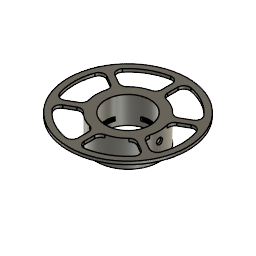
Font Reel (Autodesk Fusion 360 design; units mm, degrees)
part number: 2026-01-12-12-34-36-869
Autodesk Fusion 360 part; units mm, degrees
sketch "Sketch1" plane through (0, 0, 0) normal (0, 0, 1) x (1, 0, 0)
  circle A0 centre (0, 0) radius 90
  circle A1 centre (0, 0) radius 50
  circle A2 centre (0, 0) radius 53
  circle A3 centre (0, 0) radius 100
  line L0 (-5, 89.861) -> (-5, 52.7636)
  line L1 (5, 89.861) -> (5, 52.7636)
  line L2 (0, 110) -> (0, -110)
  line L3 (-80.3219, 40.6004) -> (-48.1946, 22.0517)
  line L4 (-75.3219, 49.2606) -> (-43.1946, 30.7119)
  line L5 (-75.3219, -49.2606) -> (-43.1946, -30.7119)
  line L6 (-80.3219, -40.6004) -> (-48.1946, -22.0517)
  line L7 (5, -89.861) -> (5, -52.7636)
  line L8 (-5, -89.861) -> (-5, -52.7636)
  line L9 (80.3219, -40.6004) -> (48.1946, -22.0517)
  line L10 (75.3219, -49.2606) -> (43.1946, -30.7119)
  line L11 (75.3219, 49.2606) -> (43.1946, 30.7119)
  line L12 (80.3219, 40.6004) -> (48.1946, 22.0517)
  circle A4 centre (0, 0) radius 40
  line L13 (-1.5, 49.9775) -> (-1.5, 39.9719)
  line L14 (1.5, 49.9775) -> (1.5, 39.9719)
  line L15 (-42.5318, 26.2878) -> (-33.8667, 21.285)
  line L16 (-44.0318, 23.6897) -> (-35.3667, 18.6869)
  line L17 (-44.0318, -23.6897) -> (-35.3667, -18.6869)
  line L18 (-42.5318, -26.2878) -> (-33.8667, -21.285)
  line L19 (-1.5, -49.9775) -> (-1.5, -39.9719)
  line L20 (1.5, -49.9775) -> (1.5, -39.9719)
  line L21 (42.5318, -26.2878) -> (33.8667, -21.285)
  line L22 (44.0318, -23.6897) -> (35.3667, -18.6869)
  line L23 (44.0318, 23.6897) -> (35.3667, 18.6869)
  line L24 (42.5318, 26.2878) -> (33.8667, 21.285)
  circle A5 centre (0, 0) radius 47
  circle A6 centre (0, 0) radius 37
  circle A7 centre (0, 0) radius 35.5
  line L25 (12.1417, 33.3591) -> (0, 0)
  line L26 (-12.1417, 33.3591) -> (0, 0)
  line L27 (12.1417, 33.3591) -> (12.6547, 34.7686)
  line L28 (-12.1417, 33.3591) -> (-12.6547, 34.7686)
  line L29 (-33.3591, 12.1417) -> (-34.7686, 12.6547)
  line L30 (-33.3591, -12.1417) -> (-34.7686, -12.6547)
  line L31 (-12.1417, -33.3591) -> (-12.6547, -34.7686)
  line L32 (12.1417, -33.3591) -> (12.6547, -34.7686)
  line L33 (33.3591, -12.1417) -> (34.7686, -12.6547)
  line L34 (33.3591, 12.1417) -> (34.7686, 12.6547)
  line L35 (-10.1986, 35.5667) -> (-9.7851, 34.1248)
  line L36 (-9.7851, 34.1248) -> (0, 0)
  line L37 (-35.5667, -10.1986) -> (-34.1248, -9.7851)
  line L38 (10.1986, -35.5667) -> (9.7851, -34.1248)
  line L39 (35.5667, 10.1986) -> (34.1248, 9.7851)
  dimension "d1" = 180
  dimension "d2" = 100
  dimension "d3" = 3
  dimension "d8" = 10
  dimension "d9" = 10
  dimension "d11" = 360
  dimension "d18" = -10
  dimension "d19" = 3
  dimension "d21" = 360
  dimension "d24" = -3
  dimension "d28" = -3
  dimension "d44" = -1.5
  dimension "d47" = 40
  dimension "d48" = 20
  dimension "d50" = 360
  dimension "d54" = 4
  dimension "d56" = 360
  constraint coincident A0.centre A1.centre
  constraint concentric A0 A1
  constraint coincident A0 L0.start
  constraint coincident A2 L0.end
  constraint vertical L0
  constraint coincident A0 L1.start
  constraint coincident A2 L1.end
  constraint parallel L0 L1
  constraint vertical L2
  constraint symmetric L0 L1 L2
  constraint coincident L2 A0.centre
  constraint coincident A1 L13.start
  constraint coincident A4 L13.end
  constraint parallel L2 L13
  constraint coincident A1 L14.start
  constraint coincident A4 L14.end
  constraint parallel L2 L14
  constraint symmetric L2 L13 L14
  constraint coincident A7 L25.start
  constraint coincident A7 L26.start
  constraint coincident A6 L27.end
  constraint parallel L25 L27
  constraint coincident A6 L28.end
  constraint parallel L26 L28
  constraint coincident A6 L35.start
  constraint coincident A7 L35.end
  measures "d1" diameter of A0
  measures "d2" diameter of A1
  measures "d9" distance of L0 L1
  measures "d19" distance of L13 L14
  measures "d47" angle of L25 L26
  measures "d48" angle of L2 L26
  measures "d54" angle of L26 L35
extrude "Extrude3" add sketch "Sketch1" along normal blind 5 contours A0 A3 L2 | A0 A2 L11 L12 | A0 A2 L9 L10 | A1 A2 L2 | A0 A2 L1 L2 | A0 A2 L2 L7 | A0 A2 L0 L2 | A0 A3 L2 | A0 A2 L2 L8 | A1 A2 L2 | A0 A2 L3 L4 | A1 L2 L13 A5 | A1 L2 L14 A5 | A0 A2 L5 L6 | A1 L2 L20 A5 | A1 L2 L19 A5 | A1 L14 L24 A5 | A1 L13 L15 A5 | L2 A4 L14 A5 | L2 A4 L13 A5 | A1 L18 L19 A5 | A1 L20 L21 A5 | L2 A4 L19 A5 | L2 A4 L20 A5 | A1 L23 L24 A5 | A4 L14 L24 A5 | A1 L15 L16 A5 | A4 L13 L15 A5 | L2 A4 A6 | L2 A4 A6 | A1 L17 L18 A5 | A4 L18 L19 A5 | A1 L21 L22 A5 | A4 L20 L21 A5 | A1 L22 L23 A5 | A4 L23 L24 A5 | A1 L16 L17 A5 | A4 L15 L16 A5 | A4 L17 L18 A5 | A4 L21 L22 A5 | A4 L22 L23 A5 | A4 L16 L17 A5
extrude "Extrude9" add sketch "Sketch1" against normal blind 40 contours A1 A2 L2 | A1 A2 L2 | A1 L2 L13 A5 | A1 L2 L14 A5 | A1 L2 L20 A5 | A1 L2 L19 A5 | L2 A4 L14 A5 | L2 A4 L13 A5 | L2 A4 L19 A5 | L2 A4 L20 A5 | A1 L23 L24 A5 | A1 L15 L16 A5 | L2 A4 A6 | L2 A4 A6 | A1 L17 L18 A5 | A1 L21 L22 A5 | A4 L23 L24 A5 | A4 L15 L16 A5 | A4 L17 L18 A5 | A4 L21 L22 A5
extrude "Extrude10" cut sketch "Sketch1" along normal blind 5 from surface at -40 contours A1 L2 L13 A5 | A1 L2 L14 A5 | A1 L2 L20 A5 | A1 L2 L19 A5 | A1 L23 L24 A5 | A1 L15 L16 A5 | A1 L17 L18 A5 | A1 L21 L22 A5
fillet "Fillet2" radius 10 24 edges at (43.1946, 30.7119, 2.5) (48.1946, 22.0517, 2.5) (48.1946, -22.0517, 2.5) (43.1946, -30.7119, 2.5) (5, -52.7636, 2.5) (-5, -52.7636, 2.5) (-43.1946, -30.7119, 2.5) (-48.1946, -22.0517, 2.5) (-48.1946, 22.0517, 2.5) (-43.1946, 30.7119, 2.5) (-5, 52.7636, 2.5) (5, 52.7636, 2.5) (75.3219, 49.2606, 2.5) (-5, 89.861, 2.5) (5, 89.861, 2.5) (-75.3219, 49.2606, 2.5) (-80.3219, 40.6004, 2.5) (-80.3219, -40.6004, 2.5) (-75.3219, -49.2606, 2.5) (-5, -89.861, 2.5) (5, -89.861, 2.5) (75.3219, -49.2606, 2.5) (80.3219, -40.6004, 2.5) (80.3219, 40.6004, 2.5)
extrude "Extrude11" add sketch "Sketch1" along normal blind 5 from surface at -29.8 contours L2 A6 A7 L27 | L2 A6 A7 L35 | L2 A6 A7 L31 | L2 A6 A7 L38 | A6 A7 L28 L35 | A6 A7 L32 L38 | A6 A7 L34 L39 | A6 A7 L30 L37 | A6 A7 L33 L39 | A6 A7 L29 L37
extrude "Extrude12" cut sketch "Sketch1" along normal blind 2 from surface at -28.3 contours L2 A6 A7 L27 | L2 A6 A7 L35 | L2 A6 A7 L31 | L2 A6 A7 L38 | A6 A7 L33 L39 | A6 A7 L29 L37
fillet "Fillet4" radius 2 6 edges at (40.7032, -23.5, -40) (40.7032, 23.5, -40) (0, 47, -40) (-40.7032, 23.5, -40) (-40.7032, -23.5, -40) (0, -47, -40)
sketch "Sketch3" plane through (0, 0, 0) normal (1, 0, 0) x (0, 1, 0)
  circle A0 centre (0, -10) radius 5
  line L0 (0, 0) -> (0, -10)
  dimension "d67" = 10
  dimension "d68" = 10
  constraint coincident L0.start origin
  constraint coincident A0.centre L0.end
  constraint vertical L0
  measures "d67" diameter of A0
  measures "d68" distance of L0.start A0.centre
extrude "Extrude15" cut sketch "Sketch3" along normal through all
